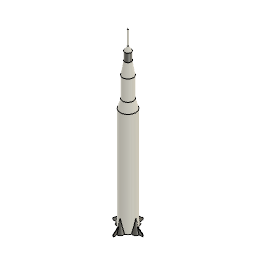
Saturn V Rocket (Autodesk Fusion 360 design; units mm, degrees)
part number: 2026-06-06-22-10-50-549
Autodesk Fusion 360 part; units mm, degrees
sketch "Sketch1" plane through (0, 0, 0) normal (0, 0, 1) x (1, 0, 0)
  circle A0 centre (0, 0) radius 27
  circle A1 centre (0, 0) radius 14.5
  dimension "d1" = 54
  dimension "d2" = 29
  constraint coincident A0.centre A1.centre
  measures "d1" diameter of A0
  measures "d2" diameter of A1
extrude "Extrude1" add sketch "Sketch1" along normal blind 360 makes body 1
sketch "Sketch2" plane through (0, 0, 360) normal (0, 0, 1) x (-1, 0, 0)
  circle A0 centre (0, 0) radius 14.5
  circle A1 centre (0, 0) radius 27
extrude "Extrude2" add sketch "Sketch2" along normal blind 30 draft -16 contours A0 | A1 bodies 1
extrude "Extrude3" add 1 faces at (-5.0343, -5.918, 390) along direction (0, 0, 1) blind 70 on bodies 1 bodies 1
extrude "Extrude4" add 1 faces at (-5.0343, -5.918, 460) along direction (0, 0, 1) blind 44 draft -9.4 on bodies 1 bodies 1
extrude "Extrude5" add 1 faces at (0.6023, -5.8536, 504) along direction (0, 0, 1) blind 28 on bodies 1 bodies 1
extrude "Extrude6" add 1 faces at (0.6023, -5.8536, 532) along direction (0, 0, 1) blind 15 draft -30.7 on bodies 1 bodies 1
extrude "Extrude7" add 1 faces at (0.7314, -0.5956, 547) along direction (0, 0, 1) blind 50 on bodies 1 bodies 1
extrude "Extrude8" add 1 faces at (0.7314, -0.5956, 597) along direction (0, 0, 1) blind 4 draft -25 on bodies 1 bodies 1
sketch "Sketch3" plane through (0, 0, 0) normal (0, 0, 1) x (1, 0, 0)
  circle A0 centre (27, 0) radius 12.5
  circle A1 centre (0, 0) radius 27
  circle A2 centre (0, 0) radius 14.5
  constraint horizontal A1.centre A0.centre
  constraint coincident A0.centre A1
  constraint tangent A0 A2
extrude "Extrude9" add sketch "Sketch3" along normal blind 45 draft -16 contours A0 A1 | A0 A1 picked at (30.9458, 2.1907) picked at (22.8179, 1.6656) bodies 1
sketch "Sketch5" plane through (0, 0, 0) normal (0, 1, 0) x (1, 0, 0)
  line L0 (27, -26) -> (27, 0)
  line L1 (27, 0) -> (52, 0)
  line L2 (52, 0) -> (52, -6)
  line L3 (52, -6) -> (27, -26)
  dimension "d21" = 26
  dimension "d22" = 25
  dimension "d23" = 6
  dimension "d24" = 27
  constraint vertical L0
  constraint perpendicular L0 L1
  constraint perpendicular L1 L2
  constraint coincident origin L1
  measures "d21" distance of L0.start L0.end
  measures "d22" distance of L0.end L1.end
  measures "d23" distance of L1.end L2.end
  measures "d24" distance of origin L0
extrude "Extrude10" add sketch "Sketch5" along normal mid plane 2 bodies 1
pattern_circular "C-Pattern1" count 4 over 360 about axis through (0, 0, 1.75) along (0, 0, 1) of "Extrude9", "Extrude10"
move_body "Move1" bodies 1 to x (1, 0, 0) y (0, 1, 0) z (0, 0, 1) at (0, 0, -300)
split "Split1" by plane through (0, 0, 0) normal (0, 0, 1) bodies 1 makes body 2 at (26.9664, -1.3458, 40)
move_body "Move2" bodies 2 1 to x (1, 0, 0) y (0, 1, 0) z (0, 0, 1) at (0, 0, 300)
combine "Combine1" operation add target body 1 tool bodies 2
named bodies: "Rocket Body"
